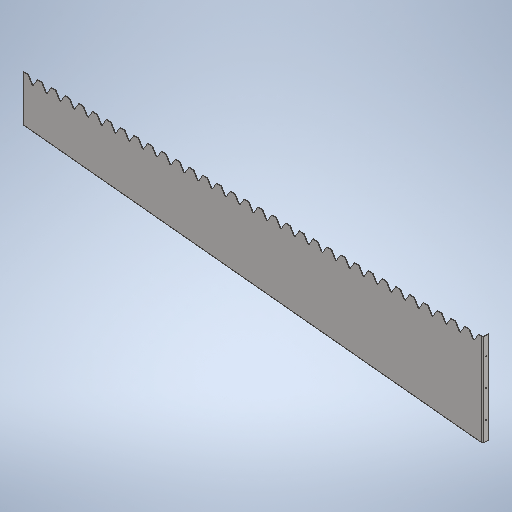
# Autodesk Inventor part: MSC 071 ridge 1
Saved by Autodesk Inventor 2025 (Build 290162010, 162A)
## iProperties
Created: 2024-06-08
Part Number: MSC 071 ridge 1
Material: Stainless Steel
Document SubType Name: Sheet Metal
Designer: admin
Density: 8 g/cm^3
Appearance: Semi-Polished
Sheet Metal Rule: AISI304 2mm Die16
Stock Number: МОО 071 гребень 1
Flat Pattern Width: 40.1115 cm
Flat Pattern Length: 205.107 cm
Flat Pattern Area: 8227.15 cm^2
Sheet Metal Width: 401,115 mm
Sheet Metal Length: 2051,070 mm
Sheet Metal Area: 822715,460 mm^2
Author: admin
Autodesk Inventor part; units mm, degrees
ref_plane "YZ Plane" through (0, 0, 0) normal (1, 0, 0) x (0, 1, 0)
ref_plane "XZ Plane" through (0, 0, 0) normal (0, 1, 0) x (-1, 0, 0)
ref_plane "XY Plane" through (0, 0, 0) normal (0, 0, 1) x (1, 0, 0)
sketch "Sketch1" plane through (0, 0, 0) normal (0, 1, 0) x (-1, 0, 0)
  line L0 (0, 0) -> (0, -400)
  line L1 (2000, -200) -> (2000, 0)
  line L2 (2000, 0) -> (0, 0)
  line L3 (0, -400) -> (10, -400)
  line L4 (2000, -200) -> (10, -400)
  dimension "d0" = 400
  dimension "d1" = 2000
  dimension "d2" = 200
  dimension "d4" = 10
  measures "d0" distance of L0.start L0.end
  measures "d1" distance of L1.end L0.start
  measures "d2" distance of L1.start L1.end
  measures "d4" distance of L0.end L3.end
extrude "Plate1" add sketch "Sketch1" along normal blind 2
sketch "Sketch3" plane through (0, 0, 0) normal (0, -1, 0) x (1, 0, 0)
  line L0 (-2000, 0) -> (0, 0) projected
  line L1 (-20, 0) -> (-37.5, -30)
  line L2 (-37.5, -30) -> (-42.5, -30)
  line L3 (-42.5, -30) -> (-60, 0)
  dimension "d12" = 5
  dimension "d13" = 40
  dimension "d14" = 30
  dimension "d15" = 20
  constraints: 6 end point, 2 point on line, 1 equal length, 1 horizontal
  measures "d12" distance of L1.end L2.end
  measures "d13" distance of L1.start L3.end
  measures "d14" distance between parallel lines of L2 L0
  measures "d15" distance of L0.end L1.start
extrude "Extrusion2" cut sketch "Sketch3" against normal through all
fillet "Fillet2" radius 2 4 edges at (-20, 1, 0) (-37.5, 1, -30) (-42.5, 1, -30) (-60, 1, 0)
pattern_linear "Rectangular Pattern1" count 33 spacing 60 along (-1, 0, 0) of "Extrusion2", "Fillet2"
sketch "Sketch4" plane through (-2, 0, 0) normal (1, 0, 0) x (0, -1, 0)
  line L0 (0, -400) -> (0, 0)
  line L1 (0, 0) -> (-25, 0)
  line L2 (-25, 0) -> (-25, -400)
  line L3 (-25, -400) -> (0, -400)
  constraints: 6 end point, 1 horizontal, 1 perpendicular, 1 vertical
edge flange "Flange1" height 25 angle 90 thickness 2 bend radius 2.75 thickness toward (1, 0, 0) relief straight relief width 2 relief depth 1 edges at (0, 0, -200) wall of the first edge with corners at (-2, 0, -400) (-2, 0, 0) (-2, 25, 0) (-2, 25, -400)
bend "Bend1"
corner "Corner1"
sketch "Sketch6" plane through (0, 25, 0) normal (1, 0, 0) x (0, 0, -1)
  circle A0 centre (80, -10) radius 2.55 projected
  circle A1 centre (385, -288.3333) radius 2.55 projected
  circle A2 centre (80, -440) radius 2.55 projected
  circle A3 centre (200, -440) radius 2.55 projected
  circle A4 centre (320, -440) radius 2.55 projected
  circle A5 centre (385, -415) radius 2.55 projected
  line L0 (0, -925) -> (30, -942.5) projected
  line L1 (30, -942.5) -> (30, -947.5) projected
  line L2 (30, -947.5) -> (0, -965) projected
  line L3 (0, -965) -> (0, -1020) projected
  arc A6 (0, -1020) -> (790, -985) centre (-511.0623, 19448.6209) ccw projected
  line L4 (790, 535) -> (790, -985) projected
  arc A7 (790, 535) -> (0, 570) centre (-511.0623, -19898.6209) ccw projected
  line L5 (0, 515) -> (0, 570) projected
  line L6 (0, 515) -> (30, 497.5) projected
  line L7 (30, 497.5) -> (30, 492.5) projected
  line L8 (30, 492.5) -> (0, 475) projected
  line L9 (0, 435) -> (0, 475) projected
  line L10 (0, 435) -> (30, 417.5) projected
  line L11 (30, 417.5) -> (30, 412.5) projected
  line L12 (30, 412.5) -> (0, 395) projected
  line L13 (0, 355) -> (0, 395) projected
  line L14 (0, 355) -> (30, 337.5) projected
  line L15 (30, 337.5) -> (30, 332.5) projected
  line L16 (30, 332.5) -> (0, 315) projected
  line L17 (0, 275) -> (0, 315) projected
  line L18 (0, 275) -> (30, 257.5) projected
  line L19 (30, 257.5) -> (30, 252.5) projected
  line L20 (30, 252.5) -> (0, 235) projected
  line L21 (0, 195) -> (0, 235) projected
  line L22 (0, 195) -> (30, 177.5) projected
  line L23 (30, 177.5) -> (30, 172.5) projected
  line L24 (30, 172.5) -> (0, 155) projected
  line L25 (0, 115) -> (0, 155) projected
  line L26 (0, 115) -> (30, 97.5) projected
  line L27 (30, 97.5) -> (30, 92.5) projected
  line L28 (30, 92.5) -> (0, 75) projected
  line L29 (0, 35) -> (0, 75) projected
  line L30 (0, 35) -> (30, 17.5) projected
  line L31 (30, 17.5) -> (30, 12.5) projected
  line L32 (30, 12.5) -> (0, -5) projected
  line L33 (0, -5) -> (0, -445) projected
  line L34 (0, -445) -> (30, -462.5) projected
  line L35 (30, -462.5) -> (30, -467.5) projected
  line L36 (30, -467.5) -> (0, -485) projected
  line L37 (0, -485) -> (0, -525) projected
  line L38 (0, -525) -> (30, -542.5) projected
  line L39 (30, -542.5) -> (30, -547.5) projected
  line L40 (30, -547.5) -> (0, -565) projected
  line L41 (0, -565) -> (0, -605) projected
  line L42 (0, -605) -> (30, -622.5) projected
  line L43 (30, -622.5) -> (30, -627.5) projected
  line L44 (30, -627.5) -> (0, -645) projected
  line L45 (0, -645) -> (0, -685) projected
  line L46 (0, -685) -> (30, -702.5) projected
  line L47 (30, -702.5) -> (30, -707.5) projected
  line L48 (30, -707.5) -> (0, -725) projected
  line L49 (0, -725) -> (0, -765) projected
  line L50 (0, -765) -> (30, -782.5) projected
  line L51 (30, -782.5) -> (30, -787.5) projected
  line L52 (30, -787.5) -> (0, -805) projected
  line L53 (0, -805) -> (0, -845) projected
  line L54 (0, -845) -> (30, -862.5) projected
  line L55 (30, -862.5) -> (30, -867.5) projected
  line L56 (30, -867.5) -> (0, -885) projected
  line L57 (0, -885) -> (0, -925) projected
  circle A8 centre (385, -161.6667) radius 2.55 projected
  circle A9 centre (385, -35) radius 2.55 projected
  circle A10 centre (320, -10) radius 2.55 projected
  circle A11 centre (200, -10) radius 2.55 projected
  circle A12 centre (80, -10) radius 2.55 projected
  line L58 (370, -25) -> (370, -425) projected
  line L59 (370, -425) -> (30, -425) projected
  line L60 (30, -25) -> (30, -425) projected
  line L61 (370, -25) -> (30, -25) projected
  circle A13 centre (320, -10) radius 2.55 projected
  point P0 (0, -25)
extrude "Extrusion3" cut sketch "Sketch6" against normal through all contours A0 | A10 | A11
equation "\"d3\" = Thickness"
equation "\"d22\" = BendReliefWidth"
equation "\"d23\" = BendReliefDepth"
equation "\"d24\" = MinimumRemnant"
equation "\"d25\" = TransitionRadius"
equation "\"d28\" = BendRadius"
equation "\"d29\" = CornerReliefSize"
equation "\"d30\" = GapSize"
equation "\"d31\" = JacobiRadiusSize"
equation "\"BendReliefWidth\" = Thickness"
equation "\"BendReliefDepth\" = 0.5 * Thickness"
equation "\"CornerReliefSize\" = 4 * Thickness"
equation "\"MinimumRemnant\" = 2 * Thickness"
equation "\"TransitionRadius\" = BendRadius"
equation "\"JacobiRadiusSize\" = BendRadius"
equation "\"GapSize\" = Thickness"
equation "\"Thickness\" = 2"
equation "\"BendRadius\" = 2.75"
body "Solid1"
